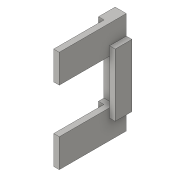
# Autodesk Inventor part: CatwalkHolder
Saved by Autodesk Inventor 2016 (Build 200138000, 138)
## iProperties
Created: 2016-11-30
Part Number: CatwalkHolder
Material: Generic
Document SubType Name: Modeling
Designer: reinert
Density: 1 g/cm^3
Appearance: Default
Author: reinert
Autodesk Inventor part; units mm, degrees
ref_plane "YZ Plane" through (0, 0, 0) normal (1, 0, 0) x (0, 1, 0)
ref_plane "XZ Plane" through (0, 0, 0) normal (0, 1, 0) x (-1, 0, 0)
ref_plane "XY Plane" through (0, 0, 0) normal (0, 0, 1) x (1, 0, 0)
sketch "Sketch1" plane through (0, 0, 0) normal (0, 1, 0) x (-1, 0, 0)
  line L0 (0, 0) -> (10, 0)
  line L1 (10, 0) -> (10, -112)
  line L2 (10, -112) -> (0, -112)
  line L3 (0, -112) -> (0, 0)
  line L4 (10, -112) -> (10, -147)
  line L5 (10, -147) -> (30, -147)
  line L6 (10, 0) -> (10, 35)
  line L7 (10, 35) -> (30, 35)
  line L8 (30, 35) -> (30, -147)
  dimension "d16" = 35
  dimension "d17" = 20
  dimension "d18" = 35
  dimension "d19" = 20
  dimension "d28" = 112
  dimension "d35" = 10
  constraints: 18 end point, 3 perpendicular, 2 parallel, 1 horizontal, 1 point on line, 1 vertical
  measures "d16" distance of L1.end L4.end
  measures "d17" distance of L4.end L5.end
  measures "d18" distance of L0.end L6.end
  measures "d19" distance of L6.end L7.end
  measures "d28" distance of L2.end L0.start
  measures "d35" distance of L0.start L0.end
extrude "Extrusion1" add sketch "Sketch1" along normal blind 30
sketch "Sketch2" plane through (0, 0, 0) normal (0, -1, 0) x (1, 0, 0)
  line L0 (-30, -147) -> (-30, 35) projected
  line L1 (-30, -96) -> (-10, -96)
  line L2 (-10, -96) -> (-10, -16)
  line L3 (-10, -16) -> (-30, -16)
  line L4 (-30, -16) -> (-30, -96)
  line L5 (-10, 0) -> (0, 0) projected
  dimension "d22" = 20
  dimension "d23" = 80
  dimension "d25" = 16
  constraints: 8 end point, 2 parallel, 1 horizontal, 1 perpendicular, 1 point on line
  measures "d22" distance of L3.end L2.end
  measures "d23" distance of L2.end L1.end
  measures "d25" distance from line of L5 L2.end
extrude "Extrusion2" cut sketch "Sketch2" against normal blind 10
sketch "Sketch3" plane through (0, 0, 0) normal (0, -1, 0) x (1, 0, 0)
  line L0 (-10, -16) -> (-10, -96) projected
  line L1 (-10, -96) -> (-20, -96)
  line L2 (-20, -96) -> (-20, -147)
  line L3 (-20, -147) -> (-10, -147)
  line L4 (-10, -147) -> (-10, -96)
  line L5 (-10, -16) -> (-20, -16)
  line L6 (-20, -16) -> (-20, 35)
  line L7 (-20, 35) -> (-10, 35)
  line L8 (-10, 35) -> (-10, -16)
  point P0 (0, 0)
  dimension "d29" = 10
  dimension "d30" = 51
  dimension "d31" = 10
  dimension "d32" = 51
  constraints: 16 end point, 4 parallel, 2 horizontal, 2 perpendicular
  measures "d29" distance of L3.end L2.end
  measures "d30" distance of L2.end L1.end
  measures "d31" distance of L6.end L7.end
  measures "d32" distance of L5.end L6.end
extrude "Extrusion3" add sketch "Sketch3" along normal blind 90
body "Solid1"
